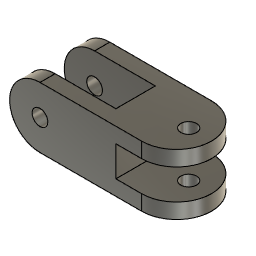
link_1 (Autodesk Fusion 360 design; units mm, degrees)
Autodesk Fusion 360 part; units mm, degrees
sketch "Sketch1" plane through (0, 0, 0) normal (0, 1, 0) x (1, 0, 0)
  circle A0 centre (0, 0) radius 2.6
  circle A1 centre (0, 0) radius 10
  line L0 (0, 0) -> (0, -10) construction
  line L1 (0, -10) -> (20, -10)
  line L2 (20, -10) -> (20, 10)
  line L3 (20, 10) -> (0, 10)
  line L4 (20, -10) -> (25, -10)
  line L5 (25, -10) -> (25, 10)
  line L6 (25, 10) -> (20, 10)
  line L7 (25, -10) -> (45, -10)
  line L8 (45, -10) -> (45, -5)
  line L9 (45, -5) -> (25, -5)
  line L10 (25, 10) -> (45, 10)
  line L11 (45, 10) -> (45, 5)
  line L12 (45, 5) -> (25, 5)
  dimension "d1" = 5.2
  dimension "d2" = 20
  dimension "d3" = 20
  dimension "d4" = 20
  dimension "d5" = 5
  dimension "d6" = 20
  dimension "d7" = 20
  dimension "d8" = 5
  dimension "d20" = 20
  dimension "d21" = 5
  constraint coincident A0.centre A1.centre
  constraint coincident A1 L0.end
  constraint vertical L0
  constraint tangent A1 L1
  constraint perpendicular L1 L2
  constraint coincident A1 L3.end
  constraint tangent A1 L3
  constraint perpendicular L2 L4
  constraint perpendicular L4 L5
  constraint perpendicular L5 L7
  constraint perpendicular L7 L8
  constraint coincident L5 L9.end
  constraint perpendicular L5 L9
  constraint perpendicular L5 L10
  constraint perpendicular L10 L11
  constraint coincident L5 L12.end
  constraint perpendicular L5 L12
  measures "d1" diameter of A0
  measures "d2" diameter of A1
  measures "d3" distance of L0.end L1.end
  measures "d4" distance of L1.end L2.end
  measures "d5" distance of L1.end L4.end
  measures "d6" distance of L4.end L5.end
  measures "d7" distance of L4.end L7.end
  measures "d8" distance of L7.end L8.end
  measures "d20" distance of L5.end L10.end
  measures "d21" distance of L10.end L11.end
extrude "Extrude1" add sketch "Sketch1" along normal blind 5 contours A1 | A1 L1 L2 L3 makes body 1
extrude "Extrude2" add sketch "Sketch1" along normal blind 5 from surface at 18 separate body contours A1 | A1 L1 L2 L3 makes body 2
extrude "Extrude3" add sketch "Sketch1" along normal blind 23 contours L2 L4 L5 L6 | L5 L10 L11 L12 | L5 L7 L8 L9 bodies 1 2
sketch "Sketch2" plane through (0, 0, 10) normal (0, 0, 1) x (-1, 0, 0)
  line L0 (0, 0) -> (-45, 0)
  line L1 (-45, 0) -> (-45, -23)
  line L2 (-45, -23) -> (0, -23)
  line L3 (0, -23) -> (0, -18)
  line L4 (0, -18) -> (-20, -18)
  line L5 (-20, -18) -> (-20, -5)
  line L6 (-20, -5) -> (0, -5)
  line L7 (0, -5) -> (0, 0)
  line L8 (-45, -11.5) -> (-37.5, -11.5) construction
  circle A0 centre (-37.5, -11.5) radius 2.6
  dimension "d17" = 7.5
  dimension "d18" = 5.2
  constraint midpoint L1 L8.start
  constraint perpendicular L1 L8
  constraint coincident L8.end A0.centre
  measures "d17" distance of L8.start L8.end
  measures "d18" diameter of A0
extrude "Extrude4" cut sketch "Sketch2" against normal through all contours A0 bodies 1
fillet "Fillet1" radius 11.5 4 edges at (45, 0, 7.5) (45, 0, -7.5) (45, 23, 7.5) (45, 23, -7.5) on bodies 1
equation "d12 = 5 mm + 13 mm"
equation "d15 = 10 mm + 13 mm"
equation "d17 = ( 15 / 2 ) * 1 mm"
equation "d23 = ( 23 / 2 ) * 1 mm"
